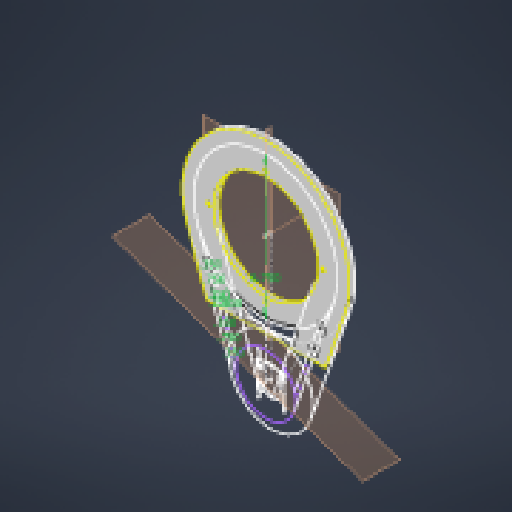
# Autodesk Inventor part: Board
Saved by Autodesk Inventor 2024 (Build 280153000, 153)
## iProperties
Created: 2023-10-21
Part Number: Board
Material: Generic
Document SubType Name: Modeling
Designer: range
Density: 1 g/cm^3
Appearance: Default
Author: range
Autodesk Inventor part; units mm, degrees
ref_plane "YZ Plane" through (0, 0, 0) normal (1, 0, 0) x (0, 1, 0)
ref_plane "XZ Plane" through (0, 0, 0) normal (0, 1, 0) x (-1, 0, 0)
ref_plane "XY Plane" through (0, 0, 0) normal (0, 0, 1) x (1, 0, 0)
ref_plane "Work Plane1" through (0, 0, 0) normal (0, 0, 1) x (1, 0, 0)
sketch "Sketch1" plane through (0, 0, 0) normal (0, 0, 1) x (1, 0, 0)
  circle A0 centre (0, -68.3) radius 2.5 projected
  circle A1 centre (-68.3, 0) radius 2.5 projected
  circle A2 centre (0, 68.3) radius 2.5 projected
  circle A3 centre (68.3, 0) radius 2.5 projected
  circle A4 centre (0, 0) radius 74.3 projected
  circle A5 centre (0, 0) radius 62.3 projected
  arc A6 (-10.8532, -157.7212) -> (10.8532, -157.7212) centre (0, -152.4) ccw construction
  circle A7 centre (0, 0) radius 79.1775 projected
  line L0 (-10.8532, -157.7212) -> (-71.0925, -34.8557) construction
  line L1 (10.8532, -157.7212) -> (71.0925, -34.8557) construction
  arc A8 (-10.8532, -157.7212) -> (10.8532, -157.7212) centre (0, -152.4) ccw
  arc A9 (71.0925, -34.8557) -> (-71.0925, -34.8557) centre (0, 0) ccw
  line L2 (0, -152.4) -> (0, 0) construction
  circle A10 centre (0, 0) radius 100
  circle A11 centre (0, -152.4) radius 50
  line L3 (-47.2324, -168.8042) -> (-94.4649, -32.8084)
  line L4 (47.2324, -168.8042) -> (94.4649, -32.8084)
  line L5 (71.1287, -100) -> (-71.1287, -100)
  line L6 (15.494, -167.894) -> (-15.494, -167.894)
  line L7 (-15.494, -167.894) -> (-15.494, -136.906)
  line L8 (-15.494, -136.906) -> (15.494, -136.906)
  line L9 (15.494, -136.906) -> (15.494, -167.894)
  line L10 (15.494, -167.894) -> (-15.494, -136.906) construction
  line L11 (-15.494, -167.894) -> (15.494, -136.906) construction
  line L12 (-15.494, -128.016) -> (-15.494, -145.796) construction
  line L13 (-16.994, -128.016) -> (-16.994, -145.796)
  line L14 (-13.994, -145.796) -> (-13.994, -128.016)
  arc A12 (-13.994, -128.016) -> (-16.994, -128.016) centre (-15.494, -128.016) ccw
  arc A13 (-16.994, -145.796) -> (-13.994, -145.796) centre (-15.494, -145.796) ccw
  line L15 (-15.494, -159.004) -> (-15.494, -176.784) construction
  line L16 (-16.994, -159.004) -> (-16.994, -176.784)
  line L17 (-13.994, -176.784) -> (-13.994, -159.004)
  arc A14 (-13.994, -159.004) -> (-16.994, -159.004) centre (-15.494, -159.004) ccw
  arc A15 (-16.994, -176.784) -> (-13.994, -176.784) centre (-15.494, -176.784) ccw
  line L18 (15.494, -145.796) -> (15.494, -128.016) construction
  line L19 (16.994, -145.796) -> (16.994, -128.016)
  line L20 (13.994, -128.016) -> (13.994, -145.796)
  arc A16 (13.994, -145.796) -> (16.994, -145.796) centre (15.494, -145.796) ccw
  arc A17 (16.994, -128.016) -> (13.994, -128.016) centre (15.494, -128.016) ccw
  line L21 (15.494, -159.004) -> (15.494, -176.784) construction
  line L22 (13.994, -159.004) -> (13.994, -176.784)
  line L23 (16.994, -176.784) -> (16.994, -159.004)
  arc A18 (16.994, -159.004) -> (13.994, -159.004) centre (15.494, -159.004) ccw
  arc A19 (13.994, -176.784) -> (16.994, -176.784) centre (15.494, -176.784) ccw
  circle A20 centre (0, -152.4) radius 11.493 construction
  line L24 (0, -146.05) -> (0, -158.75) construction
  line L25 (-11.493, -146.05) -> (-11.493, -158.75)
  line L26 (11.493, -158.75) -> (11.493, -146.05)
  arc A21 (11.493, -146.05) -> (-11.493, -146.05) centre (0, -146.05) ccw
  arc A22 (-11.493, -158.75) -> (11.493, -158.75) centre (0, -158.75) ccw
  dimension "d0" = 24.175
  dimension "d1" = 152.4
  dimension "d4" = 200
  dimension "d5" = 100
  dimension "d6" = 30.988
  dimension "d7" = 30.988
  dimension "d15" = 8.89
  dimension "d16" = 3
  dimension "d17" = 8.89
  dimension "d18" = 3
  dimension "d19" = 8.89
  dimension "d20" = 3
  dimension "d21" = 8.89
  dimension "d22" = 3
  dimension "d23" = 6.35
  constraints: 64 end point, 32 point on circle, 30 tangent, 16 centre point, 8 parallel, 7 midpoint, 4 coincident, 4 point on line, 3 vertical, 2 horizontal, 1 perpendicular, 2 other
  measures "d0" diameter of A6
  measures "d1" distance of L2.start L2.end
  measures "d4" diameter of A10
  measures "d5" diameter of A11
  measures "d6" distance of L7.end L8.end
  measures "d7" distance of L8.end L6.start
  measures "d15" distance of L7.end L12.end
  measures "d16" diameter of A13
  measures "d17" distance of L6.end L15.end
  measures "d18" diameter of A15
  measures "d19" distance of L8.end L18.end
  measures "d20" diameter of A17
  measures "d21" distance of L6.start L21.end
  measures "d22" diameter of A19
  measures "d23" distance of A20.centre L24.end
extrude "Extrusion1" add sketch "Sketch1" along normal blind 6.35 contours A4 | A7 | A10 | A10 L5 L3 | L4 L5 A10
sketch "Sketch2" plane through (0, 0, 6.35) normal (0, 0, 1) x (1, 0, 0)
  circle A0 centre (0, 0) radius 62.3 projected
  circle A1 centre (68.3, 0) radius 2.5 projected
  circle A2 centre (0, 68.3) radius 2.5 projected
  circle A3 centre (-68.3, 0) radius 2.5 projected
  circle A4 centre (0, -68.3) radius 2.5 projected
  line L0 (71.1287, -100) -> (94.4649, -32.8084) projected
  arc A5 (94.4649, -32.8084) -> (-94.4649, -32.8084) centre (0, 0) ccw projected
  line L1 (-94.4649, -32.8084) -> (-71.1287, -100) projected
  circle A6 centre (0, 0) radius 85.725
  circle A7 centre (0, -152.4) radius 35.725
  line L2 (-80.98, -28.125) -> (-33.7476, -164.1208)
  line L3 (-56.9859, -19.7917) -> (-9.7535, -155.7875)
  line L4 (0, -68.3) -> (0, -152.4)
  line L5 (80.98, -28.125) -> (33.7476, -164.1208)
  line L6 (56.9859, -19.7917) -> (9.7535, -155.7875)
  circle A8 centre (0, 0) radius 100 construction
  line L7 (-56.0172, -100) -> (56.0172, -100) construction
  line L8 (-64.3585, -56.6282) -> (-34.4196, -142.831)
  line L9 (-64.3585, -56.6282) -> (-70.357, -58.7116)
  line L10 (-34.4196, -142.831) -> (-40.4181, -144.9143)
  line L11 (-61.4419, -65.0262) -> (-67.4404, -67.1095)
  line L12 (-55.1919, -83.0217) -> (-61.1904, -85.105)
  line L13 (-52.2752, -91.4196) -> (-58.2737, -93.503)
  line L14 (-37.3363, -134.4331) -> (-43.3348, -136.5164)
  line L15 (-43.5863, -116.4375) -> (-49.5848, -118.5208)
  line L16 (-46.5029, -108.0396) -> (-52.5015, -110.1229)
  line L17 (64.3585, -56.6282) -> (34.4196, -142.831)
  line L18 (64.3585, -56.6282) -> (70.357, -58.7116)
  line L19 (34.4196, -142.831) -> (40.4181, -144.9143)
  line L20 (61.4419, -65.0262) -> (67.4404, -67.1095)
  line L21 (55.1919, -83.0217) -> (61.1904, -85.105)
  line L22 (52.2752, -91.4196) -> (58.2737, -93.503)
  line L23 (37.3363, -134.4331) -> (43.3348, -136.5164)
  line L24 (43.5863, -116.4375) -> (49.5848, -118.5208)
  line L25 (46.5029, -108.0396) -> (52.5015, -110.1229)
  line L26 (-71.1287, -100) -> (71.1287, -100) projected
  point P0 (33.7476, -164.1208)
  point P1 (80.98, -28.125)
  point P2 (37.0033, -77.3274)
  point P3 (20.9741, -123.4801)
  point P4 (-20.9741, -123.4801)
  point P5 (-37.0033, -77.3274)
  point P6 (-80.98, -28.125)
  point P7 (-33.7476, -164.1208)
  dimension "d24" = 171.45
  dimension "d26" = 25.4
  dimension "d32" = 6.35
  dimension "d33" = 8.89
  dimension "d34" = 19.05
  dimension "d35" = 8.89
  dimension "d36" = 8.89
  dimension "d37" = 19.05
  dimension "d38" = 8.89
  constraints: 48 end point, 20 symmetric about line, 9 parallel, 4 point on line, 2 coincident, 2 perpendicular, 1 centre point, 1 concentric, 1 horizontal, 1 tangent, 1 vertical, 8 other
  measures "d26" distance between parallel lines of L2 L3
  measures "d32" distance between parallel lines of L2 L8
  measures "d33" distance between parallel lines of L9 L11
  measures "d34" distance between parallel lines of L11 L12
  measures "d35" distance between parallel lines of L12 L13
  measures "d36" distance between parallel lines of L10 L14
  measures "d37" distance between parallel lines of L14 L15
  measures "d38" distance between parallel lines of L15 L16
extrude "Extrusion2" cut sketch "Sketch2" against normal through all contours A6 L4 L26 L3 | L6 L26 L4 A6 | L8 L11 L2 L9 | L26 L4 A7 L3 | L18 L5 L20 L17 | L6 A7 L4 L26 | L8 L13 L2 L12 | L10 L2 L14 L8 | L8 L15 L2 L16 | L21 L5 L22 L17 | L17 L23 L5 L19 | L25 L5 L24 L17
fillet "Fillet1" radius 1.5875 2 edges at (37.0033, -77.3274, 3.175) (-37.0033, -77.3274, 3.175)
fillet "Fillet2" radius 3.175 18 edges at (-59.732, -89.304, 6.35) (-68.8987, -62.9105, 6.35) (0, -85.725, 6.35) (-35.3745, -79.136, 6.35) (-32.46, -90.4088, 6.35) (35.3745, -79.136, 6.35) (68.8987, -62.9105, 6.35) (59.732, -89.304, 6.35) (32.46, -90.4088, 6.35) (68.8987, -62.9105, 0) (59.732, -89.304, 0) (-68.8987, -62.9105, 0) (-59.732, -89.304, 0) (-35.3745, -79.136, 0) (0, -85.725, 0) (35.3745, -79.136, 0) (32.46, -90.4088, 0) (-32.46, -90.4088, 0)
fillet "Fillet2" radius 1.5875 32 edges at (67.3578, -57.6699, 6.35) (67.3578, -57.6699, 0) (62.9002, -60.8272, 0) (62.9002, -60.8272, 6.35) (64.3585, -56.6282, 3.175) (61.4419, -65.0262, 3.175) (64.4411, -66.0678, 0) (64.4411, -66.0678, 6.35) (58.1911, -84.0634, 0) (53.7335, -87.2207, 0) (53.7335, -87.2207, 6.35) (-58.1911, -84.0634, 0) (-58.1911, -84.0634, 6.35) (-55.1919, -83.0217, 3.175) (-53.7335, -87.2207, 6.35) (-52.2752, -91.4196, 3.175) (-55.2744, -92.4613, 6.35) (-53.7335, -87.2207, 0) (-55.2744, -92.4613, 0) (-67.3578, -57.6699, 0) (-67.3578, -57.6699, 6.35) (-64.3585, -56.6282, 3.175) (-62.9002, -60.8272, 6.35) (-64.4411, -66.0678, 6.35) (-61.4419, -65.0262, 3.175) (-64.4411, -66.0678, 0) (-62.9002, -60.8272, 0) (55.2744, -92.4613, 0) (52.2752, -91.4196, 3.175) (55.1919, -83.0217, 3.175) (55.2744, -92.4613, 6.35) (58.1911, -84.0634, 6.35)
ref_plane "Work Plane2" through (47.2324, -168.8042, 6.35) normal (0.328084, 0.9446486, 0) x (0, 0, -1)
sketch "Sketch3" plane through (47.2324, -168.8042, 6.35) normal (0.328084, 0.9446486, 0) x (0, 0, -1)
  circle A0 centre (3.175, -2.3917) radius 3.975
  line L0 (6.35, 0) -> (0, 0) projected
  point P0 (6.35, 100)
  dimension "d40" = 7.95
  constraints: 2 point on circle, 1 centre point
  measures "d40" diameter of A0
extrude "Extrusion3" cut sketch "Sketch3" along normal through all both and the other way through all
ref_plane "Work Plane3" through (0, 0, 6.35) normal (1, 0, 0) x (0, 0, -1)
mirror "Mirror1" about plane through (0, 0, 6.35) normal (1, 0, 0) of "Extrusion3"
equation "\"d15\" = d19"
equation "\"d17\" = d15"
equation "\"d21\" = d17"
body "Solid1"
